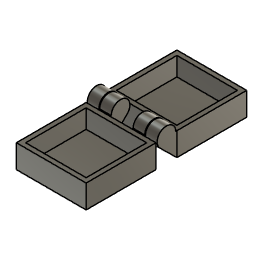
day20-box_with_hinges (Autodesk Fusion 360 design; units mm, degrees)
part number: 2025-06-29-20-21-11-885
part number: 2025-06-29-20-23-21-177
part number: 2025-06-29-20-27-52-331
Autodesk Fusion 360 part; units mm, degrees
sketch "box-width" plane through (0, 0, 0) normal (0, 0, 1) x (1, 0, 0) in component "box_bottom"
  line L0 (0, 0) -> (30, 0)
  line L1 (30, 0) -> (30, 30)
  line L2 (30, 30) -> (0, 30)
  line L3 (0, 30) -> (0, 0)
  dimension "d3" = 30
  dimension "d4" = 30
  constraint horizontal L0
  constraint vertical L1
  constraint horizontal L2
  constraint vertical L3
  constraint coincident L0.start L3.end
  measures "d3" distance of L0.start L0.end
  measures "d4" distance of L0.start L2.end
extrude "Extrude1" add sketch "box-width" along normal blind 10 makes body 1 in component "box_bottom"
shell "Shell1" thickness 2 removed faces 1 at (10, 20, 10) on bodies 1 in component "box_bottom"
sketch "box-width (2)" plane through (0, 0, 0) normal (0, 0, 1) x (1, 0, 0) in component "box_top"
  line L0 (0, 0) -> (30, 0)
  line L1 (30, 0) -> (30, 30)
  line L2 (30, 30) -> (0, 30)
  line L3 (0, 30) -> (0, 0)
  dimension "d3_1" = 30
  dimension "d4_1" = 30
  constraint horizontal L0
  constraint vertical L1
  constraint horizontal L2
  constraint vertical L3
  constraint coincident L0.start L3.end
  measures "d3_1" distance of L0.start L0.end
  measures "d4_1" distance of L0.start L2.end
extrude "Extrude1'" add sketch "box-width (2)" along normal blind 10 separate body makes body 2 in component "box_top"
shell "Shell1'" thickness 2 removed faces 1 at (10, 20, 10) on bodies 2 in component "box_top"
sketch "side_profile_hinge" plane through (0, 0, 0) normal (-1, 0, 0) x (0, -1, 0) in component "box_bottom"
  line L0 (-30, 0) -> (0, 0)
  line L1 (0, 0) -> (0, 10)
  line L2 (0, 10) -> (-30, 10)
  line L3 (-30, 10) -> (-30, 0)
  line L4 (0, 10) -> (4.5, 10)
  circle A0 centre (4.5, 10) radius 4
  line L5 (0, 0) -> (7.2976, 7.1411)
  dimension "d16" = 4.5
  dimension "d17" = 8
  constraint coincident L1.end L2.start
  constraint perpendicular L1 L4
  constraint coincident L4.end A0.centre
  constraint coincident L0.end L1.start
  constraint coincident A0 L5.end
  constraint tangent A0 L5
  measures "d16" distance of L1.end L4.end
  measures "d17" diameter of A0
extrude "Extrude2" add sketch "side_profile_hinge" against normal blind 5 separate body contours L1 L4 A0 L5 | A0 makes body 3 in component "box_bottom"
sketch "Sketch3" plane through (5, 0, 0) normal (1, 0, 0) x (0, 1, 0) in component "box_bottom"
  line L0 (0, 0) -> (0, 10)
  line L1 (0, 10) -> (-0.5, 10)
  arc A0 (-0.5, 10) -> (-7.2976, 7.1411) centre (-4.5, 10) ccw
  line L2 (-7.2976, 7.1411) -> (0, 0)
  arc A1 (-0.5, 10) -> (-7.2976, 7.1411) centre (-4.5, 10) ccw
  circle A2 centre (-4.5, 10) radius 2
  dimension "d20" = 4
  constraint concentric A0 A2
  measures "d20" diameter of A2
extrude "Extrude3" add sketch "Sketch3" along normal blind 3.8 draft -10 contours A2 bodies 3 in component "box_bottom"
fillet "Fillet1" radius 0.5 1 edges at (8.8, -5.74, 10.4809) on bodies 3 in component "box_bottom"
sketch "Sketch2" plane through (25, 0, 0) normal (-1, 0, 0) x (0, -1, 0) in component "box_top"
  line L0 (9, 0) -> (9, 10)
  line L1 (9, 10) -> (8.5, 10)
  arc A0 (8.5, 10) -> (1.7024, 7.1411) centre (4.5, 10) ccw
  line L2 (1.7024, 7.1411) -> (9, 0)
  arc A1 (8.5, 10) -> (1.7024, 7.1411) centre (4.5, 10) ccw
  line L3 (0, 0) -> (0, 10)
  circle A2 centre (4.5, 10) radius 4
  line L4 (0, 10) -> (0.5, 10)
  line L5 (0, 0) -> (7.2976, 7.1411)
  circle A3 centre (4.5, 10) radius 2
  constraint concentric A1 A2
  constraint coincident A0.end A2
  constraint coincident L3.end L4.start
  constraint coincident A1 L4.end
  constraint coincident L3.start L5.start
  constraint coincident A2 L5.end
  constraint tangent A2 L5
extrude "Extrude2'" add sketch "Sketch2" along normal blind 5 from surface at 0.3 separate body contours A0 L2 A1 L3 A2 L4 L5 | L2 A2 L5 | A0 A1 A2 | A3 makes body 4 in component "box_top"
combine "Combine2" operation cut target body 4 tool bodies 3 body 3 seen with x (-1, 0, 0) y (0, -1, 0) z (0, 0, 1) at (30, -9, 0) keep tools in component "box_top"
ref_plane "WorkPlane1" through (15, 15, 5) normal (-1, 0, 0) x (0, -1, 0) in component "box_top"
mirror "Mirror1" about plane through (15, -24, 5) normal (1, 0, 0) of bodies 3 makes body 5 in component "box_bottom"
move_face "OffsetFaces2" offset -0.2 3 faces at (24.1855, -5.4282, 8.3923) (21.2, -4.5207, 10.2757) (21.5904, -3.5748, 11.0484) on bodies 4 in component "box_top"
mirror "Mirror2" about plane through (15, 15, 5) normal (-1, 0, 0) of bodies 4 makes body 6 in component "box_top"
combine "Combine3" operation add target body 2 tool bodies 4 6 keep tools in component "box_top"
combine "Combine1" operation add target body 1 tool bodies 3 5 keep tools in component "box_bottom"
component "box_bottom" placed x (1, 0, 0) y (0, 1, 0) z (0, 0, 1) at (0, 0, 0)
component "box_top" placed x (-1, 0, 0) y (0, -1, 0) z (0, 0, 1) at (30, -9, 0)
equation "box_width = 30 mm"
equation "box_height = 20 mm"
equation "d3 = box_width"
equation "d4 = box_width"
equation "d5 = box_height / 2"
equation "wall_thickness = 2 mm"
equation "d3_1 = box_width"
equation "d4_1 = box_width"
equation "d5_1 = box_height / 2"
equation "wall_thickness_1 = 2 mm"
